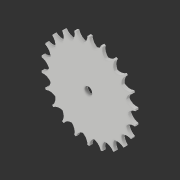
# Autodesk Inventor part: Sprocket Chain Positioning 1
Saved by Autodesk Inventor 2019 (Build 230136000, 136)
## iProperties
Created: 2020-06-02
Part Number: Sprocket Chain Positioning 1
Material: Generic
Document SubType Name: Modeling
Designer: 18186
Density: 1 g/cm^3
Appearance: Default
Author: 18186
Autodesk Inventor part; units mm, degrees
ref_plane "YZ Plane" through (0, 0, 0) normal (1, 0, 0) x (0, 1, 0)
ref_plane "XZ Plane" through (0, 0, 0) normal (0, 1, 0) x (-1, 0, 0)
ref_plane "XY Plane" through (0, 0, 0) normal (0, 0, 1) x (1, 0, 0)
sketch "Sketch1" plane through (0, 0, 0) normal (0, 0, 1) x (1, 0, 0)
  line L0 (0, 0) -> (0, 38.1) construction
  line L1 (0, 38.1) -> (0.635, 38.1)
  line L2 (0, 38.1) -> (-0.635, 38.1)
  line L3 (0.635, 38.1) -> (4.365, 38.1) construction
  line L4 (4.365, 38.1) -> (4.365, 31.5352) construction
  arc A0 (0.635, 38.1) -> (4.365, 31.5352) centre (8.2771, 38.1) ccw
  line L5 (-0.635, 38.1) -> (-4.365, 38.1) construction
  line L6 (-4.365, 38.1) -> (-4.365, 31.5352) construction
  arc A1 (-4.365, 31.5352) -> (-0.635, 38.1) centre (-8.2771, 38.1) ccw
  line L7 (-10.734, 36.5567) -> (-11.3433, 36.3778)
  line L8 (-10.734, 36.5567) -> (-10.1247, 36.7356)
  arc A2 (-10.1247, 36.7356) -> (-4.6963, 31.4875) centre (-2.7922, 38.8886) ccw
  arc A3 (-13.0727, 29.028) -> (-11.3433, 36.3778) centre (-18.6758, 34.2248) ccw
  line L9 (-20.5984, 32.0518) -> (-21.1326, 31.7085)
  line L10 (-20.5984, 32.0518) -> (-20.0642, 32.3951)
  arc A4 (-20.0642, 32.3951) -> (-13.3771, 28.889) centre (-13.6353, 36.5267) ccw
  arc A5 (-20.7213, 24.1692) -> (-21.1326, 31.7085) centre (-27.5615, 27.5768) ccw
  line L11 (-28.7941, 24.9502) -> (-29.2099, 24.4703)
  line L12 (-28.7941, 24.9502) -> (-28.3782, 25.4301)
  arc A6 (-28.3782, 25.4301) -> (-20.9742, 23.95) centre (-23.3737, 31.2056) ccw
  arc A7 (-26.6912, 17.3523) -> (-29.2099, 24.4703) centre (-34.2144, 18.6948) ccw
  line L13 (-34.657, 15.8273) -> (-34.9208, 15.2497)
  line L14 (-34.657, 15.8273) -> (-34.3932, 16.4049)
  arc A8 (-34.3932, 16.4049) -> (-26.8721, 17.0707) centre (-31.2186, 23.3564) ccw
  arc A9 (-30.4987, 9.1296) -> (-34.9208, 15.2497) centre (-38.0954, 8.2982) ccw
  line L15 (-37.7122, 5.4222) -> (-37.8026, 4.7937)
  line L16 (-37.7122, 5.4222) -> (-37.6218, 6.0507)
  arc A10 (-37.6218, 6.0507) -> (-30.593, 8.8085) centre (-36.5342, 13.615) ccw
  arc A11 (-31.8354, 0.1673) -> (-37.8026, 4.7937) centre (-38.8901, -2.7706) ccw
  line L17 (-37.7122, -5.4222) -> (-37.6218, -6.0507)
  line L18 (-37.7122, -5.4222) -> (-37.8026, -4.7937)
  arc A12 (-37.8026, -4.7937) -> (-31.8354, -0.1673) centre (-38.8901, 2.7706) ccw
  arc A13 (-30.593, -8.8085) -> (-37.6218, -6.0507) centre (-36.5342, -13.615) ccw
  line L19 (-34.657, -15.8273) -> (-34.3932, -16.4049)
  line L20 (-34.657, -15.8273) -> (-34.9208, -15.2497)
  arc A14 (-34.9208, -15.2497) -> (-30.4987, -9.1296) centre (-38.0954, -8.2982) ccw
  arc A15 (-26.8721, -17.0707) -> (-34.3932, -16.4049) centre (-31.2186, -23.3564) ccw
  line L21 (-28.7941, -24.9502) -> (-28.3782, -25.4301)
  line L22 (-28.7941, -24.9502) -> (-29.2099, -24.4703)
  arc A16 (-29.2099, -24.4703) -> (-26.6912, -17.3523) centre (-34.2144, -18.6948) ccw
  arc A17 (-20.9742, -23.95) -> (-28.3782, -25.4301) centre (-23.3737, -31.2056) ccw
  line L23 (-20.5984, -32.0518) -> (-20.0642, -32.3951)
  line L24 (-20.5984, -32.0518) -> (-21.1326, -31.7085)
  arc A18 (-21.1326, -31.7085) -> (-20.7213, -24.1692) centre (-27.5615, -27.5768) ccw
  arc A19 (-13.3771, -28.889) -> (-20.0642, -32.3951) centre (-13.6353, -36.5267) ccw
  line L25 (-10.734, -36.5567) -> (-10.1247, -36.7356)
  line L26 (-10.734, -36.5567) -> (-11.3433, -36.3778)
  arc A20 (-11.3433, -36.3778) -> (-13.0727, -29.028) centre (-18.6758, -34.2248) ccw
  arc A21 (-4.6963, -31.4875) -> (-10.1247, -36.7356) centre (-2.7922, -38.8886) ccw
  line L27 (0, -38.1) -> (0.635, -38.1)
  line L28 (0, -38.1) -> (-0.635, -38.1)
  arc A22 (-0.635, -38.1) -> (-4.365, -31.5352) centre (-8.2771, -38.1) ccw
  arc A23 (4.365, -31.5352) -> (0.635, -38.1) centre (8.2771, -38.1) ccw
  line L29 (10.734, -36.5567) -> (11.3433, -36.3778)
  line L30 (10.734, -36.5567) -> (10.1247, -36.7356)
  arc A24 (10.1247, -36.7356) -> (4.6963, -31.4875) centre (2.7922, -38.8886) ccw
  arc A25 (13.0727, -29.028) -> (11.3433, -36.3778) centre (18.6758, -34.2248) ccw
  line L31 (20.5984, -32.0518) -> (21.1326, -31.7085)
  line L32 (20.5984, -32.0518) -> (20.0642, -32.3951)
  arc A26 (20.0642, -32.3951) -> (13.3771, -28.889) centre (13.6353, -36.5267) ccw
  arc A27 (20.7213, -24.1692) -> (21.1326, -31.7085) centre (27.5615, -27.5768) ccw
  line L33 (28.7941, -24.9502) -> (29.2099, -24.4703)
  line L34 (28.7941, -24.9502) -> (28.3782, -25.4301)
  arc A28 (28.3782, -25.4301) -> (20.9742, -23.95) centre (23.3737, -31.2056) ccw
  arc A29 (26.6912, -17.3523) -> (29.2099, -24.4703) centre (34.2144, -18.6948) ccw
  line L35 (34.657, -15.8273) -> (34.9208, -15.2497)
  line L36 (34.657, -15.8273) -> (34.3932, -16.4049)
  arc A30 (34.3932, -16.4049) -> (26.8721, -17.0707) centre (31.2186, -23.3564) ccw
  arc A31 (30.4987, -9.1296) -> (34.9208, -15.2497) centre (38.0954, -8.2982) ccw
  line L37 (37.7122, -5.4222) -> (37.8026, -4.7937)
  line L38 (37.7122, -5.4222) -> (37.6218, -6.0507)
  arc A32 (37.6218, -6.0507) -> (30.593, -8.8085) centre (36.5342, -13.615) ccw
  arc A33 (31.8354, -0.1673) -> (37.8026, -4.7937) centre (38.8901, 2.7706) ccw
  line L39 (37.7122, 5.4222) -> (37.6218, 6.0507)
  line L40 (37.7122, 5.4222) -> (37.8026, 4.7937)
  arc A34 (37.8026, 4.7937) -> (31.8354, 0.1673) centre (38.8901, -2.7706) ccw
  arc A35 (30.593, 8.8085) -> (37.6218, 6.0507) centre (36.5342, 13.615) ccw
  line L41 (34.657, 15.8273) -> (34.3932, 16.4049)
  line L42 (34.657, 15.8273) -> (34.9208, 15.2497)
  arc A36 (34.9208, 15.2497) -> (30.4987, 9.1296) centre (38.0954, 8.2982) ccw
  arc A37 (26.8721, 17.0707) -> (34.3932, 16.4049) centre (31.2186, 23.3564) ccw
  line L43 (28.7941, 24.9502) -> (28.3782, 25.4301)
  line L44 (28.7941, 24.9502) -> (29.2099, 24.4703)
  arc A38 (29.2099, 24.4703) -> (26.6912, 17.3523) centre (34.2144, 18.6948) ccw
  arc A39 (20.9742, 23.95) -> (28.3782, 25.4301) centre (23.3737, 31.2056) ccw
  line L45 (20.5984, 32.0518) -> (20.0642, 32.3951)
  line L46 (20.5984, 32.0518) -> (21.1326, 31.7085)
  arc A40 (21.1326, 31.7085) -> (20.7213, 24.1692) centre (27.5615, 27.5768) ccw
  arc A41 (13.3771, 28.889) -> (20.0642, 32.3951) centre (13.6353, 36.5267) ccw
  arc A42 (-4.365, 31.5352) -> (-4.6963, 31.4875) centre (0, 0) ccw
  arc A43 (-13.0727, 29.028) -> (-13.3771, 28.889) centre (0, 0) ccw
  arc A44 (-20.7213, 24.1692) -> (-20.9742, 23.95) centre (0, 0) ccw
  arc A45 (-26.6912, 17.3523) -> (-26.8721, 17.0707) centre (0, 0) ccw
  arc A46 (-30.4987, 9.1296) -> (-30.593, 8.8085) centre (0, 0) ccw
  arc A47 (-31.8354, 0.1673) -> (-31.8354, -0.1673) centre (0, 0) ccw
  arc A48 (-30.593, -8.8085) -> (-30.4987, -9.1296) centre (0, 0) ccw
  arc A49 (-26.8721, -17.0707) -> (-26.6912, -17.3523) centre (0, 0) ccw
  arc A50 (-20.9742, -23.95) -> (-20.7213, -24.1692) centre (0, 0) ccw
  arc A51 (-13.3771, -28.889) -> (-13.0727, -29.028) centre (0, 0) ccw
  arc A52 (-4.6963, -31.4875) -> (-4.365, -31.5352) centre (0, 0) ccw
  arc A53 (4.365, -31.5352) -> (4.6963, -31.4875) centre (0, 0) ccw
  arc A54 (13.0727, -29.028) -> (13.3771, -28.889) centre (0, 0) ccw
  arc A55 (20.7213, -24.1692) -> (20.9742, -23.95) centre (0, 0) ccw
  arc A56 (26.6912, -17.3523) -> (26.8721, -17.0707) centre (0, 0) ccw
  arc A57 (30.4987, -9.1296) -> (30.593, -8.8085) centre (0, 0) ccw
  arc A58 (31.8354, -0.1673) -> (31.8354, 0.1673) centre (0, 0) ccw
  arc A59 (30.593, 8.8085) -> (30.4987, 9.1296) centre (0, 0) ccw
  arc A60 (26.8721, 17.0707) -> (26.6912, 17.3523) centre (0, 0) ccw
  arc A61 (20.9742, 23.95) -> (20.7213, 24.1692) centre (0, 0) ccw
  line L47 (10.734, 36.5567) -> (10.1247, 36.7356)
  line L48 (10.734, 36.5567) -> (11.3433, 36.3778)
  arc A62 (11.3433, 36.3778) -> (13.0727, 29.028) centre (18.6758, 34.2248) ccw
  arc A63 (4.6963, 31.4875) -> (10.1247, 36.7356) centre (2.7922, 38.8886) ccw
  arc A64 (4.6963, 31.4875) -> (4.365, 31.5352) centre (0, 0) ccw
  arc A65 (13.3771, 28.889) -> (13.0727, 29.028) centre (0, 0) ccw
  arc A66 (20.9742, 23.95) -> (20.7213, 24.1692) centre (0, 0) ccw
  arc A67 (26.8721, 17.0707) -> (26.6912, 17.3523) centre (0, 0) ccw
  arc A68 (30.593, 8.8085) -> (30.4987, 9.1296) centre (0, 0) ccw
  arc A69 (31.8354, -0.1673) -> (31.8354, 0.1673) centre (0, 0) ccw
  arc A70 (30.4987, -9.1296) -> (30.593, -8.8085) centre (0, 0) ccw
  arc A71 (26.6912, -17.3523) -> (26.8721, -17.0707) centre (0, 0) ccw
  arc A72 (20.7213, -24.1692) -> (20.9742, -23.95) centre (0, 0) ccw
  arc A73 (13.0727, -29.028) -> (13.3771, -28.889) centre (0, 0) ccw
  arc A74 (4.365, -31.5352) -> (4.6963, -31.4875) centre (0, 0) ccw
  arc A75 (-4.6963, -31.4875) -> (-4.365, -31.5352) centre (0, 0) ccw
  arc A76 (-20.9742, -23.95) -> (-20.7213, -24.1692) centre (0, 0) ccw
  arc A77 (-13.3771, -28.889) -> (-13.0727, -29.028) centre (0, 0) ccw
  arc A78 (-26.8721, -17.0707) -> (-26.6912, -17.3523) centre (0, 0) ccw
  arc A79 (-30.593, -8.8085) -> (-30.4987, -9.1296) centre (0, 0) ccw
  arc A80 (-31.8354, 0.1673) -> (-31.8354, -0.1673) centre (0, 0) ccw
  arc A81 (-30.4987, 9.1296) -> (-30.593, 8.8085) centre (0, 0) ccw
  arc A82 (-26.6912, 17.3523) -> (-26.8721, 17.0707) centre (0, 0) ccw
  arc A83 (-20.7213, 24.1692) -> (-20.9742, 23.95) centre (0, 0) ccw
  arc A84 (-4.365, 31.5352) -> (-4.6963, 31.4875) centre (0, 0) ccw
  arc A85 (-13.0727, 29.028) -> (-13.3771, 28.889) centre (0, 0) ccw
  dimension "d2" = 38.1
  dimension "d3" = 0.635
  dimension "d4" = 0.635
  dimension "d5" = 3.73
  dimension "d8" = 360
  constraints: 172 point on circle, 98 end point, 86 centre point, 3 horizontal, 2 coincident, 2 line through centre, 2 symmetric about line, 2 vertical, 242 other
  measures "d2" distance of L0.start L0.end
  measures "d3" distance of L0.end L1.end
  measures "d4" distance of L0.end L2.end
  measures "d5" distance of L1.end L3.end
extrude "Extrusion1" add sketch "Sketch1" along normal blind 2.54
sketch "Sketch2" plane through (0, 0, 2.54) normal (0, 0, 1) x (1, 0, 0)
  circle A0 centre (0, 0) radius 3.175
  dimension "d12" = 6.35
  constraints: 1 centre point, 1 coincident
  measures "d12" diameter of A0
extrude "Extrusion2" cut sketch "Sketch2" against normal blind 25.4
body "Solid1"
